Autodesk Fusion 360 part; units mm, degrees
(part 4 of 7)
sketch "Sketch83" plane through (0, 0, 14.6) normal (0, 0, -1) x (1, 0, 0)
  line L0 (95.9, -25.9) -> (101.9, -25.9)
  line L1 (95.9, -24.9) -> (95.9, -25.9)
  line L2 (126.4, -65.1) -> (125.4, -65.1)
  line L3 (106.4, -85.1) -> (106.4, -84.1)
  line L4 (106.4, -75.1) -> (106.4, -72.4023)
  line L5 (113.7023, -65.1) -> (116.4, -65.1)
  line L6 (116.4, -65.1) -> (113.7023, -65.1)
  line L7 (113.7023, -65.1) -> (114.7023, -65.1)
  line L8 (113.7023, -65.1) -> (114.7023, -65.1)
  line L9 (124.3722, -66.1) -> (115.1419, -66.1)
  line L10 (125.4, -65.1) -> (125.4, -59.1)
  line L11 (124.4, -65.1) -> (124.4, -60.1)
  line L12 (125.4, -59.1) -> (124.4, -59.1)
  arc A0 (106.4, -84.1) -> (125.4, -65.1) centre (106.4, -65.1) ccw
  arc A1 (106.4, -72.4023) -> (113.7023, -65.1) centre (106.4, -65.1) ccw
  arc A2 (109.2557, -72.8958) -> (114.1671, -68.0326) centre (106.4, -65.1) ccw
  line L13 (125.4, -65.1) -> (126.4, -65.1)
  line L14 (106.4, -73.4023) -> (106.4, -72.4023)
  line L15 (107.4, -74.049) -> (107.4, -83.0722)
  line L16 (106.4, -84.1) -> (100.4, -84.1)
  line L17 (100.4, -84.1) -> (100.4, -83.1)
  line L18 (101.4, -83.1) -> (106.4, -83.1)
  line L19 (106.4, -85.1) -> (106.4, -84.1)
  line L20 (100.4, -83.1) -> (106.4, -77.1)
  line L21 (101.4, -83.1) -> (108.8853, -83.1) construction
  line L22 (101.4, -83.1) -> (106.4, -78.1)
  line L23 (101.4, -83.1) -> (108.4711, -83.1) construction
  line L24 (106.4, -83.1) -> (106.4, -78.1)
  line L25 (106.4, -77.1) -> (106.4, -72.4023)
  line L26 (106.4, -83.1) -> (106.4, -78.1)
  line L27 (106.4, -77.1) -> (106.4, -75.1)
  line L28 (124.4, -59.1) -> (118.4, -65.1)
  line L29 (124.4, -59.1) -> (132.8853, -59.1) construction
  line L30 (119.4, -65.1) -> (124.4, -60.1)
  line L31 (119.4, -65.1) -> (126.4711, -65.1) construction
  line L32 (113.7023, -65.1) -> (118.4, -65.1)
  line L33 (119.4, -65.1) -> (124.4, -65.1)
  line L34 (124.4, -65.1) -> (119.4, -65.1)
  line L35 (118.4, -65.1) -> (114.7023, -65.1)
  line L36 (115.1419, -66.1) -> (125.3631, -66.1) construction
  line L37 (115.1419, -66.1) -> (122.396, -73.3541)
  line L38 (115.1419, -66.1) -> (125.8031, -66.1) construction
  line L39 (115.1106, -67.0687) -> (121.5189, -73.477)
  line L40 (121.5189, -73.477) -> (115.1106, -67.0687)
  arc A3 (122.396, -73.3541) -> (124.3722, -66.1) centre (106.4, -65.1) ccw
  line L41 (110.8485, -77.4975) -> (107.4, -74.049)
  line L42 (111.5557, -76.7904) -> (108.6326, -73.8674)
  line L43 (108.6326, -73.8674) -> (114.9008, -80.1355)
  line L44 (107.4, -74.049) -> (114.517, -81.166)
  arc A4 (107.4, -83.0722) -> (114.517, -81.166) centre (106.4, -65.1) ccw
  arc A5 (115.9173, -80.3781) -> (121.7571, -74.4894) centre (106.4, -65.1) ccw
  line L45 (115.7249, -77.2044) -> (115.9173, -80.3781)
  line L46 (114.7267, -77.2649) -> (114.9008, -80.1355)
  line L47 (117.5062, -74.2879) -> (121.7571, -74.4894)
  line L48 (117.5535, -73.2891) -> (121.5189, -73.477)
  line L49 (121.7571, -74.4894) -> (115.5425, -74.1949)
  line L50 (114.5378, -74.1472) -> (108.6326, -73.8674)
  line L51 (121.5189, -73.477) -> (115.4816, -73.1909)
  line L52 (114.4769, -73.1432) -> (109.2557, -72.8958)
  line L53 (115.9173, -80.3781) -> (115.5425, -74.1949)
  line L54 (115.4816, -73.1909) -> (115.1106, -67.0687)
  line L55 (114.9008, -80.1355) -> (114.5378, -74.1472)
  line L56 (114.4769, -73.1432) -> (114.1671, -68.0326)
  line L57 (27.2, 4.5) -> (66.7, 4.5)
  line L58 (46.95, 4.5) -> (46.95, -21.9501) construction
  line L59 (-13.5, -74.049) -> (-20.617, -81.166)
  line L60 (-14.7326, -73.8674) -> (-21.0008, -80.1355)
  circle A6 centre (-16.25, -62.1) radius 2.5
  line L61 (-12.5, -77.1) -> (-12.5, -75.1)
  arc A7 (-20.2671, -68.0326) -> (-15.3557, -72.8958) centre (-12.5, -65.1) ccw
  line L62 (-12.5, -73.4023) -> (-12.5, -72.4023)
  line L63 (-22.0173, -80.3781) -> (-21.6425, -74.1949)
  line L64 (-31.5, -59.1) -> (-30.5, -59.1)
  line L65 (-21.2419, -66.1) -> (-31.9031, -66.1) construction
  line L66 (-16.9485, -77.4975) -> (-13.5, -74.049)
  line L67 (-22.5, -65.1) -> (-19.8023, -65.1)
  line L68 (-20.5769, -73.1432) -> (-20.2671, -68.0326)
  arc A8 (-32.5, -65.1) -> (-12.5, -85.1) centre (-12.5, -65.1) ccw
  line L69 (-20.5769, -73.1432) -> (-15.3557, -72.8958)
  arc A9 (-19.8023, -65.1) -> (-12.5, -72.4023) centre (-12.5, -65.1) ccw
  arc A10 (-31.5, -65.1) -> (-12.5, -84.1) centre (-12.5, -65.1) ccw
  line L70 (-20.6378, -74.1472) -> (-14.7326, -73.8674)
  arc A11 (-20.617, -81.166) -> (-13.5, -83.0722) centre (-12.5, -65.1) ccw
  line L71 (-12.5, -85.1) -> (-12.5, -84.1)
  line L72 (-21.2106, -67.0687) -> (-27.6189, -73.477)
  line L73 (-25.5, -65.1) -> (-30.5, -65.1)
  line L74 (-19.8023, -65.1) -> (-24.5, -65.1)
  line L75 (-27.8571, -74.4894) -> (-21.6425, -74.1949)
  line L76 (-25.5, -65.1) -> (-30.5, -60.1)
  line L77 (-19.8023, -65.1) -> (-20.8023, -65.1)
  line L78 (-30.4722, -66.1) -> (-21.2419, -66.1)
  arc A12 (-27.8571, -74.4894) -> (-22.0173, -80.3781) centre (-12.5, -65.1) ccw
  arc A13 (-30.4722, -66.1) -> (-28.496, -73.3541) centre (-12.5, -65.1) ccw
  line L79 (-21.2419, -66.1) -> (-31.4631, -66.1) construction
  line L80 (-7.5, -83.1) -> (-14.5711, -83.1) construction
  line L81 (-13.5, -74.049) -> (-13.5, -83.0722)
  line L82 (-25.5, -65.1) -> (-32.5711, -65.1) construction
  line L83 (-30.5, -65.1) -> (-30.5, -60.1)
  line L84 (-6.5, -83.1) -> (-12.5, -77.1)
  line L85 (-21.0008, -80.1355) -> (-20.6378, -74.1472)
  line L86 (-12.5, -75.1) -> (-12.5, -72.4023)
  line L87 (-23.6062, -74.2879) -> (-27.8571, -74.4894)
  line L88 (-19.8023, -65.1) -> (-22.5, -65.1)
  line L89 (-31.5, -65.1) -> (-32.5, -65.1)
  line L90 (-12.5, -83.1) -> (-12.5, -78.1)
  line L91 (-17.6557, -76.7904) -> (-14.7326, -73.8674)
  line L92 (-7.5, -83.1) -> (-14.9853, -83.1) construction
  line L93 (-7.5, -83.1) -> (-12.5, -83.1)
  line L94 (-6.5, -84.1) -> (-6.5, -83.1)
  line L95 (-24.5, -65.1) -> (-20.8023, -65.1)
  line L96 (-12.5, -85.1) -> (-12.5, -84.1)
  line L97 (-21.8249, -77.2044) -> (-22.0173, -80.3781)
  line L98 (-12.5, -77.1) -> (-12.5, -72.4023)
  line L99 (-12.5, -84.1) -> (-6.5, -84.1)
  line L100 (-7.5, -83.1) -> (-12.5, -78.1)
  line L101 (-12.5, -83.1) -> (-12.5, -78.1)
  line L102 (-27.6189, -73.477) -> (-21.2106, -67.0687)
  line L103 (-20.8267, -77.2649) -> (-21.0008, -80.1355)
  line L104 (-30.5, -65.1) -> (-25.5, -65.1)
  line L105 (-30.5, -59.1) -> (-38.9853, -59.1) construction
  line L106 (-21.5816, -73.1909) -> (-21.2106, -67.0687)
  line L107 (-23.6535, -73.2891) -> (-27.6189, -73.477)
  line L108 (-32.5, -65.1) -> (-31.5, -65.1)
  line L109 (-27.6189, -73.477) -> (-21.5816, -73.1909)
  line L110 (-30.5, -59.1) -> (-24.5, -65.1)
  line L111 (-19.8023, -65.1) -> (-20.8023, -65.1)
  line L112 (-31.5, -65.1) -> (-31.5, -59.1)
  line L113 (-21.2419, -66.1) -> (-28.496, -73.3541)
  line L114 (101.9, -25.9) -> (101.9, -24.9)
  line L115 (101.9, -24.9) -> (95.9, -24.9)
  dimension "d560" = 1
  dimension "d561" = 1
  dimension "d562" = 1
  dimension "d563" = 1
  dimension "d566" = 6
  dimension "d567" = 6
  dimension "d569" = 6
  dimension "d570" = 1
  dimension "d571" = 45
  dimension "d572" = 1
  dimension "d573" = 45
  dimension "d574" = 135
  dimension "d575" = 1
  dimension "d576" = 45
  dimension "d580" = 45
  dimension "d583" = 1
  dimension "d585" = 1
  constraint parallel L4 L19
  constraint parallel L5 L7
  constraint concentric A1 A2
  constraint perpendicular L10 L32
  constraint coincident L14.start L19
  constraint coincident L4.end L19
  constraint collinear L13 L32
  constraint coincident L5.end L32
  constraint parallel L14 L19
  constraint perpendicular L3 L16
  constraint perpendicular L16 L17
  constraint collinear L19 L24
  constraint coincident L4.start L19
  constraint horizontal L21
  constraint coincident L20.end L26
  constraint horizontal L23
  constraint collinear L24 L25
  constraint collinear L26 L27
  constraint horizontal L29
  constraint horizontal L31
  constraint collinear L32 L33
  constraint collinear L34 L35
  constraint horizontal L36
  constraint horizontal L38
  constraint parallel L39 L40
  constraint concentric A3 A4
  constraint parallel L42 L43
  constraint parallel L41 L44
  constraint concentric A4 A5
  constraint parallel L46 L55
  constraint parallel L48 L51
  constraint collinear L49 L50
  constraint coincident L52.start L55
  constraint collinear L51 L52
  constraint coincident L51.end L53
  constraint collinear L53 L54
  constraint collinear L55 L56
  constraint midpoint L57 L58.start
  constraint perpendicular L57 L58
  constraint symmetric L3.start L58 A8.end
  constraint symmetric L2.start L58 A8.start
  constraint symmetric L2.end L58 A10.start
  constraint symmetric L3.end L58 A10.end
  constraint symmetric L18.end L58 L90.start
  constraint symmetric L4.start L58 L61.end
  constraint symmetric L5.end L58 L67.start
  constraint symmetric L5.start L58 L67.end
  constraint symmetric L7.end L58 L77.end
  constraint symmetric L11.start L58 L73.end
  constraint symmetric L10.end L58 L64.start
  constraint symmetric L12.end L58 L64.end
  constraint symmetric A0 L58 A10
  constraint symmetric L14.start L58 L62.start
  constraint symmetric L4.end L58 L62.end
  constraint symmetric A1 L58 A9
  constraint symmetric A2 L58 A7
  constraint symmetric L9.start L58 L78.start
  constraint symmetric L15.end L58 A11.end
  constraint symmetric L16.end L58 L94.start
  constraint symmetric L17.end L58 L84.start
  constraint symmetric L20.end L58 L61.start
  constraint symmetric L21.end L58 L92.end
  constraint symmetric L18.start L58 L80.start
  constraint symmetric L22.end L58 L90.end
  constraint symmetric L23.end L58 L80.end
  constraint symmetric L28.end L58 L74.end
  constraint symmetric L29.end L58 L105.end
  constraint symmetric L30.start L58 L73.start
  constraint symmetric L11.end L58 L76.end
  constraint symmetric L31.end L58 L82.end
  constraint symmetric L36.end L58 L79.end
  constraint symmetric L9.end L58 L65.start
  constraint symmetric L38.end L58 L65.end
  constraint symmetric L37.end L58 A13.end
  constraint symmetric A3 L58 A13
  constraint symmetric L42.start L58 L91.start
  constraint symmetric L41.start L58 L66.start
  constraint symmetric L44.end L58 L59.end
  constraint symmetric A4 L58 A11
  constraint symmetric A5 L58 A12
  constraint symmetric L15.start L58 L59.start
  constraint symmetric L46.start L58 L103.start
  constraint symmetric L45.start L58 L97.start
  constraint symmetric L47.start L58 L87.start
  constraint symmetric L48.start L58 L107.start
  constraint symmetric L43.end L58 L60.end
  constraint symmetric A5.start L58 L63.start
  constraint symmetric L49.end L58 L63.end
  constraint symmetric L52.start L58 L68.start
  constraint symmetric L50.start L58 L70.start
  constraint symmetric L51.end L58 L106.start
  constraint symmetric A2.end L58 A7.start
  constraint symmetric L39.start L58 L72.start
  constraint symmetric L42.end L58 L60.start
  constraint symmetric A2.start L58 A7.end
  constraint symmetric A5.end L58 L75.start
  constraint symmetric L39.end L58 L72.end
  measures "d560" distance of L2.start L2.end
  measures "d561" distance of L3.start L3.end
  measures "d562" distance of L3.end L18.end
  measures "d563" distance of L5.start L7.end
  measures "d566" distance of L2.end L10.end
  measures "d567" distance of L11.start L12.end
  measures "d569" distance of L3.end L16.end
  measures "d570" distance of L16.end L17.end
  measures "d571" angle of L20 L21
  measures "d572" distance of L17.end L18.start
  measures "d573" angle of L22 L23
  measures "d574" angle of L28 L29
  measures "d575" distance of L28.end L30.start
  measures "d576" angle of L30 L31
  measures "d580" angle of L37 L38
  measures "d583" distance of L42.start L41.start
  measures "d585" distance of L46.start L45.start
extrude "Extrude70" add sketch "Sketch83" along normal blind 1 contours L4 L5 L6 L7 L8 L10 L12 A0 A1 L14 L16 L17 L20 L25 L27 L28 L32 L35 | L61 L62 L64 L67 A9 A10 L74 L77 L84 L86 L88 L94 L95 L98 L99 L110 L111 L112 bodies 3 6
sketch "Sketch86" plane through (0, 0, 15.6) normal (0, 0, 1) x (-1, 0, 0)
  line L0 (29.1144, 32.8) -> (-123.0144, 32.8)
  arc A0 (-123.0144, 32.8) -> (-126.4, 25.3) centre (-116.4, 25.3) ccw
  line L1 (-126.4, 25.3) -> (-126.4, -65.1)
  arc A1 (-126.4, -65.1) -> (-106.4, -85.1) centre (-106.4, -65.1) ccw
  line L2 (-106.4, -85.1) -> (12.5, -85.1)
  arc A2 (12.5, -85.1) -> (32.5, -65.1) centre (12.5, -65.1) ccw
  line L3 (32.5, -65.1) -> (32.5, -25.2)
  line L4 (32.5, -25.2) -> (32.5, 25.3)
  arc A3 (32.5, 25.3) -> (29.1144, 32.8) centre (22.5, 25.3) ccw
  line L5 (13, -32.2) -> (19.5, -32.2)
  line L6 (19.5, -32.2) -> (19.5, -38.2)
  line L7 (19.5, -38.2) -> (25.5, -38.2)
  line L8 (25.5, -38.2) -> (25.5, -44.7)
  line L9 (25.5, -44.7) -> (19.5, -44.7)
  line L10 (19.5, -44.7) -> (19.5, -50.7)
  line L11 (19.5, -50.7) -> (13, -50.7)
  line L12 (13, -50.7) -> (13, -44.7)
  line L13 (13, -44.7) -> (7, -44.7)
  line L14 (7, -44.7) -> (7, -38.2)
  line L15 (7, -38.2) -> (13, -38.2)
  line L16 (13, -38.2) -> (13, -32.2)
  line L17 (-34.2, 32.4) -> (-34.2, 30.4)
  line L18 (-34.2, 30.4) -> (-27.2, 30.4)
  line L19 (-27.2, 30.4) -> (-27.2, 10)
  arc A4 (-29.2, 8) -> (-27.2, 10) centre (-29.2, 10) ccw
  line L20 (-29.2, 8) -> (-64.7, 8)
  arc A5 (-66.7, 10) -> (-64.7, 8) centre (-64.7, 10) ccw
  line L21 (-66.7, 10) -> (-66.7, 30.4)
  line L22 (-66.7, 30.4) -> (-59.7, 30.4)
  line L23 (-59.7, 30.4) -> (-59.7, 32.4)
  line L24 (-59.7, 32.4) -> (-34.2, 32.4)
  arc A6 (5, 10.7) -> (5.0004, 12.7) centre (5, 11.7) ccw
  line L25 (5, 10.7) -> (-5, 10.7)
  arc A7 (-5.0004, 12.7) -> (-5, 10.7) centre (-5, 11.7) ccw
  line L26 (-5.0004, 12.7) -> (5.0004, 12.7)
  arc A8 (5.0004, 26.7) -> (5, 28.7) centre (5, 27.7) ccw
  line L27 (5.0004, 26.7) -> (-4.9996, 26.7)
  arc A9 (-5, 28.7) -> (-4.9996, 26.7) centre (-5, 27.7) ccw
  line L28 (-5, 28.7) -> (5, 28.7)
  line L29 (-8.1652, 24.7) -> (8.1652, 24.7)
  arc A10 (8.1652, 22.7) -> (8.1652, 24.7) centre (8.1652, 23.7) ccw
  line L30 (8.1652, 22.7) -> (-8.1652, 22.7)
  arc A11 (-8.1652, 24.7) -> (-8.1652, 22.7) centre (-8.1652, 23.7) ccw
  arc A12 (9, 18.7) -> (9, 20.7) centre (9, 19.7) ccw
  line L31 (9, 18.7) -> (-9, 18.7)
  arc A13 (-9, 20.7) -> (-9, 18.7) centre (-9, 19.7) ccw
  line L32 (-9, 20.7) -> (9, 20.7)
  line L33 (8.1652, 14.7) -> (-8.1652, 14.7)
  arc A14 (-8.1652, 16.7) -> (-8.1652, 14.7) centre (-8.1652, 15.7) ccw
  line L34 (-8.1652, 16.7) -> (8.1652, 16.7)
  arc A15 (8.1652, 14.7) -> (8.1652, 16.7) centre (8.1652, 15.7) ccw
  arc A16 (-102.9, 20.7) -> (-102.9, 18.7) centre (-102.9, 19.7) ccw
  line L35 (-102.9, 20.7) -> (-84.9, 20.7)
  arc A17 (-84.9, 18.7) -> (-84.9, 20.7) centre (-84.9, 19.7) ccw
  line L36 (-84.9, 18.7) -> (-102.9, 18.7)
  arc A18 (-98.9, 28.7) -> (-98.9004, 26.7) centre (-98.9, 27.7) ccw
  line L37 (-98.9, 28.7) -> (-88.9, 28.7)
  arc A19 (-88.8996, 26.7) -> (-88.9, 28.7) centre (-88.9, 27.7) ccw
  line L38 (-88.8996, 26.7) -> (-98.9004, 26.7)
  arc A20 (-102.0652, 24.7) -> (-102.0652, 22.7) centre (-102.0652, 23.7) ccw
  line L39 (-102.0652, 24.7) -> (-85.7348, 24.7)
  arc A21 (-85.7348, 22.7) -> (-85.7348, 24.7) centre (-85.7348, 23.7) ccw
  line L40 (-85.7348, 22.7) -> (-102.0652, 22.7)
  line L41 (-85.7348, 14.7) -> (-102.0652, 14.7)
  arc A22 (-102.0652, 16.7) -> (-102.0652, 14.7) centre (-102.0652, 15.7) ccw
  line L42 (-102.0652, 16.7) -> (-85.7348, 16.7)
  arc A23 (-85.7348, 14.7) -> (-85.7348, 16.7) centre (-85.7348, 15.7) ccw
  line L43 (-98.8996, 12.7) -> (-88.8996, 12.7)
  arc A24 (-88.9, 10.7) -> (-88.8996, 12.7) centre (-88.9, 11.7) ccw
  line L44 (-88.9, 10.7) -> (-98.9, 10.7)
  arc A25 (-98.8996, 12.7) -> (-98.9, 10.7) centre (-98.9, 11.7) ccw
  arc A26 (-46.45, -79.6) -> (-47.45, -79.6) centre (-46.95, -79.6) ccw
  line L45 (-46.45, -79.6) -> (-45.65, -79.6)
  arc A27 (-45.65, -80.6) -> (-45.65, -79.6) centre (-45.65, -80.1) ccw
  line L46 (-45.65, -80.6) -> (-46.45, -80.6)
  arc A28 (-47.45, -80.6) -> (-46.45, -80.6) centre (-46.95, -80.6) ccw
  line L47 (-47.45, -80.6) -> (-48.25, -80.6)
  arc A29 (-48.25, -79.6) -> (-48.25, -80.6) centre (-48.25, -80.1) ccw
  line L48 (-48.25, -79.6) -> (-47.45, -79.6)
  circle A30 centre (-110.15, -48.95) radius 3.85
  circle A31 centre (-117.65, -41.45) radius 3.85
  circle A32 centre (-102.65, -41.45) radius 3.85
  circle A33 centre (-110.15, -33.95) radius 3.85
  circle A34 centre (-117.6453, -56.4453) radius 2.35
  circle A35 centre (-102.6547, -56.4453) radius 2.35
  line L49 (0, 4.1) -> (0, -75.1)
  line L50 (0, -75.1) -> (-93.9, -75.1)
  line L51 (-93.9, -75.1) -> (-93.9, 4.1)
  line L52 (-93.9, 4.1) -> (0, 4.1)
  circle A36 centre (10.8119, -62.3239) radius 1.5
  dimension "d597" = 3
  measures "d597" diameter of A36
sketch "Sketch87" plane through (0, 0, 14.6) normal (0, 0, -1) x (1, 0, 0)
  arc A0 (-31.5, -65.1) -> (-12.5, -84.1) centre (-12.5, -65.1) ccw
  line L0 (-31.5, -65.1) -> (-31.5, -59.1)
  line L1 (-31.5, -59.1) -> (-30.5, -59.1)
  line L2 (-30.5, -59.1) -> (-24.5, -65.1)
  line L3 (-24.5, -65.1) -> (-19.8023, -65.1)
  arc A1 (-19.8023, -65.1) -> (-12.5, -72.4023) centre (-12.5, -65.1) ccw
  line L4 (-12.5, -72.4023) -> (-12.5, -77.1)
  line L5 (-12.5, -77.1) -> (-6.5, -83.1)
  line L6 (-6.5, -83.1) -> (-6.5, -84.1)
  line L7 (-6.5, -84.1) -> (-12.5, -84.1)
  line L8 (-14, -21.7213) -> (-14, -21.5571)
  arc A2 (-18.6299, -19.9) -> (-14, -21.5571) centre (-16.1626, -20.3028) ccw
  line L9 (-18.6299, -19.9) -> (-18.6563, -19.9)
  arc A3 (-18.6098, -19.7916) -> (-18.6563, -19.9) centre (-16.3363, -20.8316) ccw
  arc A4 (-13.8891, -21.3427) -> (-18.6098, -19.7916) centre (-16.1626, -20.3028) ccw
  arc A5 (-14, -21.7213) -> (-13.8891, -21.3427) centre (-16.3363, -20.8316) ccw
  circle A6 centre (-16.25, -62.1) radius 2.5
  arc A7 (-9.5307, -48.3426) -> (-9.5307, -34.5574) centre (-10.1676, -41.45) ccw
  arc A8 (-22.9827, -48.1827) -> (-9.5307, -48.3426) centre (-16.25, -47.7) ccw
  arc A9 (-22.9827, -34.7173) -> (-22.9827, -48.1827) centre (-22.5, -41.45) ccw
  arc A10 (-9.5307, -34.5574) -> (-22.9827, -34.7173) centre (-16.25, -35.2) ccw
  line L10 (-2, -24.9) -> (-8, -24.9)
  line L11 (-8, -24.9) -> (-8, -7.9)
  line L12 (-8, -7.9) -> (-13, -7.9)
  line L13 (-13, -7.9) -> (-13, -13.9)
  line L14 (-13, -13.9) -> (-25, -13.9)
  line L15 (-25, -13.9) -> (-25, -24.9)
  line L16 (-25, -24.9) -> (-30.5, -24.9)
  line L17 (-30.5, -24.9) -> (-30.5, -25.9)
  line L18 (-30.5, -25.9) -> (-31.5, -25.9)
  line L19 (-31.5, -25.9) -> (-31.5, 4.1)
  line L20 (-31.5, 4.1) -> (-32.5, 4.1)
  line L21 (-32.5, 4.1) -> (-32.5, -25.2)
  line L22 (-32.5, -25.2) -> (-32.5, -65.1)
  arc A11 (-32.5, -65.1) -> (-12.5, -85.1) centre (-12.5, -65.1) ccw
  line L23 (-12.5, -85.1) -> (-2, -85.1)
  line L24 (-2, -85.1) -> (-2, -24.9)
  line L25 (-5, -75) -> (-6, -75)
  line L26 (-6, -75) -> (-6, -57)
  line L27 (-6, -57) -> (-5, -57)
  line L28 (-5, -57) -> (-5, -75)
  line L29 (-27.5, -62.1) -> (-28.5, -62.1)
  line L30 (-28.5, -62.1) -> (-28.5, -52.1)
  line L31 (-28.5, -52.1) -> (-27.5, -52.1)
  line L32 (-27.5, -52.1) -> (-27.5, -62.1)
  dimension "d602" = 1
  dimension "d603" = 10
  constraint horizontal L25
  constraint vertical L26
  constraint horizontal L27
  constraint vertical L28
  constraint horizontal L29
  constraint vertical L30
  constraint horizontal L31
  constraint vertical L32
  constraint midpoint L2 L29.start
  measures "d602" distance of L29.start L29.end
  measures "d603" distance of L29.start L31.end
extrude "Extrude72" add sketch "Sketch87" along normal blind 1 contours L2 L30 L31 L32 | L25 L26 L27 L28 bodies 3 6 8
extrude "Extrude73" cut sketch "Sketch86" against normal blind 1 contours A36 bodies 3
sketch "Sketch88" plane through (0, 0, 15.6) normal (0, 0, 1) x (-1, 0, 0)
  circle A0 centre (10.8119, -62.3239) radius 1.5
  line L0 (29.1144, 32.8) -> (-123.0144, 32.8)
  arc A1 (-123.0144, 32.8) -> (-126.4, 25.3) centre (-116.4, 25.3) ccw
  line L1 (-126.4, 25.3) -> (-126.4, -65.1)
  arc A2 (-126.4, -65.1) -> (-106.4, -85.1) centre (-106.4, -65.1) ccw
  line L2 (-106.4, -85.1) -> (12.5, -85.1)
  arc A3 (12.5, -85.1) -> (32.5, -65.1) centre (12.5, -65.1) ccw
  line L3 (32.5, -65.1) -> (32.5, -25.2)
  line L4 (32.5, -25.2) -> (32.5, 25.3)
  arc A4 (32.5, 25.3) -> (29.1144, 32.8) centre (22.5, 25.3) ccw
  line L5 (13, -32.2) -> (19.5, -32.2)
  line L6 (19.5, -32.2) -> (19.5, -38.2)
  line L7 (19.5, -38.2) -> (25.5, -38.2)
  line L8 (25.5, -38.2) -> (25.5, -44.7)
  line L9 (25.5, -44.7) -> (19.5, -44.7)
  line L10 (19.5, -44.7) -> (19.5, -50.7)
  line L11 (19.5, -50.7) -> (13, -50.7)
  line L12 (13, -50.7) -> (13, -44.7)
  line L13 (13, -44.7) -> (7, -44.7)
  line L14 (7, -44.7) -> (7, -38.2)
  line L15 (7, -38.2) -> (13, -38.2)
  line L16 (13, -38.2) -> (13, -32.2)
  line L17 (-34.2, 32.4) -> (-34.2, 30.4)
  line L18 (-34.2, 30.4) -> (-27.2, 30.4)
  line L19 (-27.2, 30.4) -> (-27.2, 10)
  arc A5 (-29.2, 8) -> (-27.2, 10) centre (-29.2, 10) ccw
  line L20 (-29.2, 8) -> (-64.7, 8)
  arc A6 (-66.7, 10) -> (-64.7, 8) centre (-64.7, 10) ccw
  line L21 (-66.7, 10) -> (-66.7, 30.4)
  line L22 (-66.7, 30.4) -> (-59.7, 30.4)
  line L23 (-59.7, 30.4) -> (-59.7, 32.4)
  line L24 (-59.7, 32.4) -> (-34.2, 32.4)
  arc A7 (5, 10.7) -> (5.0004, 12.7) centre (5, 11.7) ccw
  line L25 (5, 10.7) -> (-5, 10.7)
  arc A8 (-5.0004, 12.7) -> (-5, 10.7) centre (-5, 11.7) ccw
  line L26 (-5.0004, 12.7) -> (5.0004, 12.7)
  arc A9 (5.0004, 26.7) -> (5, 28.7) centre (5, 27.7) ccw
  line L27 (5.0004, 26.7) -> (-4.9996, 26.7)
  arc A10 (-5, 28.7) -> (-4.9996, 26.7) centre (-5, 27.7) ccw
  line L28 (-5, 28.7) -> (5, 28.7)
  line L29 (-8.1652, 24.7) -> (8.1652, 24.7)
  arc A11 (8.1652, 22.7) -> (8.1652, 24.7) centre (8.1652, 23.7) ccw
  line L30 (8.1652, 22.7) -> (-8.1652, 22.7)
  arc A12 (-8.1652, 24.7) -> (-8.1652, 22.7) centre (-8.1652, 23.7) ccw
  arc A13 (9, 18.7) -> (9, 20.7) centre (9, 19.7) ccw
  line L31 (9, 18.7) -> (-9, 18.7)
  arc A14 (-9, 20.7) -> (-9, 18.7) centre (-9, 19.7) ccw
  line L32 (-9, 20.7) -> (9, 20.7)
  line L33 (8.1652, 14.7) -> (-8.1652, 14.7)
  arc A15 (-8.1652, 16.7) -> (-8.1652, 14.7) centre (-8.1652, 15.7) ccw
  line L34 (-8.1652, 16.7) -> (8.1652, 16.7)
  arc A16 (8.1652, 14.7) -> (8.1652, 16.7) centre (8.1652, 15.7) ccw
  arc A17 (-102.9, 20.7) -> (-102.9, 18.7) centre (-102.9, 19.7) ccw
  line L35 (-102.9, 20.7) -> (-84.9, 20.7)
  arc A18 (-84.9, 18.7) -> (-84.9, 20.7) centre (-84.9, 19.7) ccw
  line L36 (-84.9, 18.7) -> (-102.9, 18.7)
  arc A19 (-98.9, 28.7) -> (-98.9004, 26.7) centre (-98.9, 27.7) ccw
  line L37 (-98.9, 28.7) -> (-88.9, 28.7)
  arc A20 (-88.8996, 26.7) -> (-88.9, 28.7) centre (-88.9, 27.7) ccw
  line L38 (-88.8996, 26.7) -> (-98.9004, 26.7)
  arc A21 (-102.0652, 24.7) -> (-102.0652, 22.7) centre (-102.0652, 23.7) ccw
  line L39 (-102.0652, 24.7) -> (-85.7348, 24.7)
  arc A22 (-85.7348, 22.7) -> (-85.7348, 24.7) centre (-85.7348, 23.7) ccw
  line L40 (-85.7348, 22.7) -> (-102.0652, 22.7)
  line L41 (-85.7348, 14.7) -> (-102.0652, 14.7)
  arc A23 (-102.0652, 16.7) -> (-102.0652, 14.7) centre (-102.0652, 15.7) ccw
  line L42 (-102.0652, 16.7) -> (-85.7348, 16.7)
  arc A24 (-85.7348, 14.7) -> (-85.7348, 16.7) centre (-85.7348, 15.7) ccw
  line L43 (-98.8996, 12.7) -> (-88.8996, 12.7)
  arc A25 (-88.9, 10.7) -> (-88.8996, 12.7) centre (-88.9, 11.7) ccw
  line L44 (-88.9, 10.7) -> (-98.9, 10.7)
  arc A26 (-98.8996, 12.7) -> (-98.9, 10.7) centre (-98.9, 11.7) ccw
  arc A27 (-46.45, -79.6) -> (-47.45, -79.6) centre (-46.95, -79.6) ccw
  line L45 (-46.45, -79.6) -> (-45.65, -79.6)
  arc A28 (-45.65, -80.6) -> (-45.65, -79.6) centre (-45.65, -80.1) ccw
  line L46 (-45.65, -80.6) -> (-46.45, -80.6)
  arc A29 (-47.45, -80.6) -> (-46.45, -80.6) centre (-46.95, -80.6) ccw
  line L47 (-47.45, -80.6) -> (-48.25, -80.6)
  arc A30 (-48.25, -79.6) -> (-48.25, -80.6) centre (-48.25, -80.1) ccw
  line L48 (-48.25, -79.6) -> (-47.45, -79.6)
  circle A31 centre (-110.15, -48.95) radius 3.85
  circle A32 centre (-117.65, -41.45) radius 3.85
  circle A33 centre (-102.65, -41.45) radius 3.85
  circle A34 centre (-110.15, -33.95) radius 3.85
  circle A35 centre (-117.6453, -56.4453) radius 2.35
  circle A36 centre (-102.6547, -56.4453) radius 2.35
  line L49 (0, 4.1) -> (0, -75.1)
  line L50 (0, -75.1) -> (-93.9, -75.1)
  line L51 (-93.9, -75.1) -> (-93.9, 4.1)
  line L52 (-93.9, 4.1) -> (0, 4.1)
  arc A37 (-47.4908, -77.2) -> (-46.4092, -77.2) centre (-46.95, -80.1) ccw
  line L53 (-46.95, -80.1) -> (-34.95, -80.1) construction
  line L54 (-34.95, -80.1) -> (-34.95, -78.1) construction
  line L55 (-34.95, -80.1) -> (-34.95, -82.1) construction
  line L56 (-34.95, -79.1) -> (-34.95, -81.1)
  line L57 (-34.95, -81.1) -> (-35.95, -81.1)
  line L58 (-35.95, -81.1) -> (-36.95, -80.1)
  line L59 (-35.95, -81.1) -> (-34.5358, -81.1) construction
  line L60 (-36.95, -80.1) -> (-37.95, -81.1)
  line L61 (-37.95, -81.1) -> (-38.95, -81.1)
  line L62 (-38.95, -81.1) -> (-38.95, -79.1)
  line L63 (-34.95, -79.1) -> (-35.95, -79.1)
  line L64 (-35.95, -79.1) -> (-35.95, -80.1)
  line L65 (-35.95, -80.1) -> (-36.95, -79.1)
  line L66 (-36.95, -79.1) -> (-37.95, -80.1)
  line L67 (-37.95, -80.1) -> (-37.95, -79.1)
  line L68 (-37.95, -79.1) -> (-38.95, -79.1)
  line L69 (-38.95, -81.1) -> (-39.55, -81.1) construction
  line L70 (-39.55, -81.1) -> (-39.55, -79.1)
  line L71 (-39.55, -79.1) -> (-40.55, -79.1)
  line L72 (-39.55, -81.1) -> (-40.55, -81.1)
  line L73 (-40.55, -81.1) -> (-40.55, -79.1)
  line L74 (-40.95, -80.1) -> (-41.05, -80.1) construction
  line L75 (-41.05, -80.1) -> (-42.05, -80.1)
  line L76 (-42.05, -80.1) -> (-42.05, -81.1) construction
  line L77 (-42.05, -81.1) -> (-42.05, -79.1) construction
  arc A38 (-42.05, -81.1) -> (-42.05, -79.1) centre (-42.05, -80.1) ccw
  line L78 (-42.05, -81.1) -> (-42.55, -81.1)
  line L79 (-42.05, -79.1) -> (-42.55, -79.1)
  line L80 (-42.55, -79.1) -> (-42.55, -79.6)
  line L81 (-42.55, -81.1) -> (-42.55, -80.6)
  line L82 (-42.05, -80.1) -> (-42.55, -80.1)
  arc A39 (-42.55, -80.6) -> (-42.55, -79.6) centre (-42.55, -80.1) ccw
  dimension "d604" = 12
  dimension "d605" = 2
  dimension "d606" = 2
  dimension "d607" = 1
  dimension "d608" = 135
  dimension "d609" = 1
  dimension "d610" = 1
  dimension "d611" = 0.6
  dimension "d612" = 1
  dimension "d613" = 0.1
  dimension "d614" = 1
  dimension "d615" = 0.5
  dimension "d616" = 0.5
  dimension "d617" = 0.5
  dimension "d618" = 0.5
  dimension "d619" = 0.5
  constraint coincident A37.centre L53.start
  constraint parallel L45 L53
  constraint perpendicular L53 L54
  constraint perpendicular L53 L55
  constraint midpoint L54 L56.start
  constraint midpoint L55 L56.end
  constraint perpendicular L55 L57
  constraint horizontal L59
  constraint coincident L53 L58.end
  constraint perpendicular L58 L60
  constraint parallel L53 L61
  constraint perpendicular L53 L62
  constraint perpendicular L54 L63
  constraint coincident L53 L64.end
  constraint perpendicular L53 L64
  constraint parallel L58 L65
  constraint coincident L53 L66.end
  constraint perpendicular L65 L66
  constraint perpendicular L53 L67
  constraint perpendicular L62 L68
  constraint perpendicular L62 L69
  constraint perpendicular L68 L70
  constraint perpendicular L70 L71
  constraint perpendicular L70 L72
  constraint perpendicular L71 L73
  constraint midpoint L53 L74.start
  constraint perpendicular L73 L74
  constraint parallel L53 L75
  constraint coincident L75.end L76.start
  constraint coincident L74.end A38
  constraint perpendicular L53 L76
  constraint perpendicular L53 L77
  constraint perpendicular L76 L78
  constraint perpendicular L77 L79
  constraint perpendicular L79 L80
  constraint perpendicular L78 L81
  constraint perpendicular L81 L82
  constraint coincident L82.end A39.centre
  constraint coincident L75.end A39
  measures "d604" distance of A37.centre L53.end
  measures "d605" distance of L53.end L54.end
  measures "d606" distance of L53.end L55.end
  measures "d607" distance of L56.end L57.end
  measures "d608" angle of L58 L59
  measures "d609" distance of L60.end L61.end
  measures "d610" distance of L56.start L63.end
  measures "d611" distance of L61.end L69.end
  measures "d612" distance of L70.end L71.end
  measures "d613" distance of L74.start L74.end
  measures "d614" distance of L74.end L75.end
  measures "d615" distance of L76.end L78.end
  measures "d616" distance of L77.end L79.end
  measures "d617" distance of L79.end L80.end
  measures "d618" distance of L78.end L81.end
  measures "d619" distance of L75.end L82.end
sketch "icon1" plane through (0, 0, 15.6) normal (0, 0, 1) x (-1, 0, 0)
  circle A0 centre (10.8119, -62.3239) radius 1.5
  line L0 (29.1144, 32.8) -> (-123.0144, 32.8)
  arc A1 (-123.0144, 32.8) -> (-126.4, 25.3) centre (-116.4, 25.3) ccw
  line L1 (-126.4, 25.3) -> (-126.4, -65.1)
  arc A2 (-126.4, -65.1) -> (-106.4, -85.1) centre (-106.4, -65.1) ccw
  line L2 (-106.4, -85.1) -> (12.5, -85.1)
  arc A3 (12.5, -85.1) -> (32.5, -65.1) centre (12.5, -65.1) ccw
  line L3 (32.5, -65.1) -> (32.5, -25.2)
  line L4 (32.5, -25.2) -> (32.5, 25.3)
  arc A4 (32.5, 25.3) -> (29.1144, 32.8) centre (22.5, 25.3) ccw
  line L5 (13, -32.2) -> (19.5, -32.2)
  line L6 (19.5, -32.2) -> (19.5, -38.2)
  line L7 (19.5, -38.2) -> (25.5, -38.2)
  line L8 (25.5, -38.2) -> (25.5, -44.7)
  line L9 (25.5, -44.7) -> (19.5, -44.7)
  line L10 (19.5, -44.7) -> (19.5, -50.7)
  line L11 (19.5, -50.7) -> (13, -50.7)
  line L12 (13, -50.7) -> (13, -44.7)
  line L13 (13, -44.7) -> (7, -44.7)
  line L14 (7, -44.7) -> (7, -38.2)
  line L15 (7, -38.2) -> (13, -38.2)
  line L16 (13, -38.2) -> (13, -32.2)
  line L17 (-34.2, 32.4) -> (-34.2, 30.4)
  line L18 (-34.2, 30.4) -> (-27.2, 30.4)
  line L19 (-27.2, 30.4) -> (-27.2, 10)
  arc A5 (-29.2, 8) -> (-27.2, 10) centre (-29.2, 10) ccw
  line L20 (-29.2, 8) -> (-64.7, 8)
  arc A6 (-66.7, 10) -> (-64.7, 8) centre (-64.7, 10) ccw
  line L21 (-66.7, 10) -> (-66.7, 30.4)
  line L22 (-66.7, 30.4) -> (-59.7, 30.4)
  line L23 (-59.7, 30.4) -> (-59.7, 32.4)
  line L24 (-59.7, 32.4) -> (-34.2, 32.4)
  arc A7 (5, 10.7) -> (5.0004, 12.7) centre (5, 11.7) ccw
  line L25 (5, 10.7) -> (-5, 10.7)
  arc A8 (-5.0004, 12.7) -> (-5, 10.7) centre (-5, 11.7) ccw
  line L26 (-5.0004, 12.7) -> (5.0004, 12.7)
  arc A9 (5.0004, 26.7) -> (5, 28.7) centre (5, 27.7) ccw
  line L27 (5.0004, 26.7) -> (-4.9996, 26.7)
  arc A10 (-5, 28.7) -> (-4.9996, 26.7) centre (-5, 27.7) ccw
  line L28 (-5, 28.7) -> (5, 28.7)
  line L29 (-8.1652, 24.7) -> (8.1652, 24.7)
  arc A11 (8.1652, 22.7) -> (8.1652, 24.7) centre (8.1652, 23.7) ccw
  line L30 (8.1652, 22.7) -> (-8.1652, 22.7)
  arc A12 (-8.1652, 24.7) -> (-8.1652, 22.7) centre (-8.1652, 23.7) ccw
  arc A13 (9, 18.7) -> (9, 20.7) centre (9, 19.7) ccw
  line L31 (9, 18.7) -> (-9, 18.7)
  arc A14 (-9, 20.7) -> (-9, 18.7) centre (-9, 19.7) ccw
  line L32 (-9, 20.7) -> (9, 20.7)
  line L33 (8.1652, 14.7) -> (-8.1652, 14.7)
  arc A15 (-8.1652, 16.7) -> (-8.1652, 14.7) centre (-8.1652, 15.7) ccw
  line L34 (-8.1652, 16.7) -> (8.1652, 16.7)
  arc A16 (8.1652, 14.7) -> (8.1652, 16.7) centre (8.1652, 15.7) ccw
  arc A17 (-102.9, 20.7) -> (-102.9, 18.7) centre (-102.9, 19.7) ccw
  line L35 (-102.9, 20.7) -> (-84.9, 20.7)
  arc A18 (-84.9, 18.7) -> (-84.9, 20.7) centre (-84.9, 19.7) ccw
  line L36 (-84.9, 18.7) -> (-102.9, 18.7)
  arc A19 (-98.9, 28.7) -> (-98.9004, 26.7) centre (-98.9, 27.7) ccw
  line L37 (-98.9, 28.7) -> (-88.9, 28.7)
  arc A20 (-88.8996, 26.7) -> (-88.9, 28.7) centre (-88.9, 27.7) ccw
  line L38 (-88.8996, 26.7) -> (-98.9004, 26.7)
  arc A21 (-102.0652, 24.7) -> (-102.0652, 22.7) centre (-102.0652, 23.7) ccw
  line L39 (-102.0652, 24.7) -> (-85.7348, 24.7)
  arc A22 (-85.7348, 22.7) -> (-85.7348, 24.7) centre (-85.7348, 23.7) ccw
  line L40 (-85.7348, 22.7) -> (-102.0652, 22.7)
  line L41 (-85.7348, 14.7) -> (-102.0652, 14.7)
  arc A23 (-102.0652, 16.7) -> (-102.0652, 14.7) centre (-102.0652, 15.7) ccw
  line L42 (-102.0652, 16.7) -> (-85.7348, 16.7)
  arc A24 (-85.7348, 14.7) -> (-85.7348, 16.7) centre (-85.7348, 15.7) ccw
  line L43 (-98.8996, 12.7) -> (-88.8996, 12.7)
  arc A25 (-88.9, 10.7) -> (-88.8996, 12.7) centre (-88.9, 11.7) ccw
  line L44 (-88.9, 10.7) -> (-98.9, 10.7)
  arc A26 (-98.8996, 12.7) -> (-98.9, 10.7) centre (-98.9, 11.7) ccw
  arc A27 (-46.45, -79.6) -> (-47.45, -79.6) centre (-46.95, -79.6) ccw
  line L45 (-46.45, -79.6) -> (-45.65, -79.6)
  arc A28 (-45.65, -80.6) -> (-45.65, -79.6) centre (-45.65, -80.1) ccw
  line L46 (-45.65, -80.6) -> (-46.45, -80.6)
  arc A29 (-47.45, -80.6) -> (-46.45, -80.6) centre (-46.95, -80.6) ccw
  line L47 (-47.45, -80.6) -> (-48.25, -80.6)
  arc A30 (-48.25, -79.6) -> (-48.25, -80.6) centre (-48.25, -80.1) ccw
  line L48 (-48.25, -79.6) -> (-47.45, -79.6)
  circle A31 centre (-110.15, -48.95) radius 3.85
  circle A32 centre (-117.65, -41.45) radius 3.85
  circle A33 centre (-102.65, -41.45) radius 3.85
  circle A34 centre (-110.15, -33.95) radius 3.85
  circle A35 centre (-117.6453, -56.4453) radius 2.35
  circle A36 centre (-102.6547, -56.4453) radius 2.35
  line L49 (0, 4.1) -> (0, -75.1)
  line L50 (0, -75.1) -> (-93.9, -75.1)
  line L51 (-93.9, -75.1) -> (-93.9, 4.1)
  line L52 (-93.9, 4.1) -> (0, 4.1)
  circle A37 centre (16, 30.9) radius 0.4
  line L53 (15.744, 30.5926) -> (16.4, 29.8)
  line L54 (16.4, 29.8) -> (16.5662, 29.9375)
  line L55 (16.5662, 29.9375) -> (16, 30.6217)
  line L56 (16.5662, 29.9375) -> (16.8018, 29.6528)
  line L57 (16.8018, 29.6528) -> (16.0141, 29.4807)
  line L58 (16.0141, 29.4807) -> (16.4, 29.8)
  line L59 (16.0919, 31.9806) -> (16.0919, 32.8)
  line L60 (16.0919, 32.8) -> (16.0919, 31.8676)
  line L61 (16.0919, 32.8) -> (17.2457, 31.2867)
  arc A38 (16.0919, 31.8676) -> (17.2457, 31.2867) centre (16.072, 30.3917) ccw
  constraint coincident A37 L53.start
  constraint perpendicular L53 L54
  constraint perpendicular L54 L55
  constraint perpendicular L54 L56
  constraint perpendicular L56 L58
  constraint coincident L0 L59.end
  constraint perpendicular L0 L59
  constraint perpendicular L0 L60
  constraint tangent L61 A38
sketch "icon2" plane through (0, 0, 15.6) normal (0, 0, 1) x (-1, 0, 0)
  circle A0 centre (10.8119, -62.3239) radius 1.5
  line L0 (29.1144, 32.8) -> (-123.0144, 32.8)
  arc A1 (-123.0144, 32.8) -> (-126.4, 25.3) centre (-116.4, 25.3) ccw
  line L1 (-126.4, 25.3) -> (-126.4, -65.1)
  arc A2 (-126.4, -65.1) -> (-106.4, -85.1) centre (-106.4, -65.1) ccw
  line L2 (-106.4, -85.1) -> (12.5, -85.1)
  arc A3 (12.5, -85.1) -> (32.5, -65.1) centre (12.5, -65.1) ccw
  line L3 (32.5, -65.1) -> (32.5, -25.2)
  line L4 (32.5, -25.2) -> (32.5, 25.3)
  arc A4 (32.5, 25.3) -> (29.1144, 32.8) centre (22.5, 25.3) ccw
  line L5 (13, -32.2) -> (19.5, -32.2)
  line L6 (19.5, -32.2) -> (19.5, -38.2)
  line L7 (19.5, -38.2) -> (25.5, -38.2)
  line L8 (25.5, -38.2) -> (25.5, -44.7)
  line L9 (25.5, -44.7) -> (19.5, -44.7)
  line L10 (19.5, -44.7) -> (19.5, -50.7)
  line L11 (19.5, -50.7) -> (13, -50.7)
  line L12 (13, -50.7) -> (13, -44.7)
  line L13 (13, -44.7) -> (7, -44.7)
  line L14 (7, -44.7) -> (7, -38.2)
  line L15 (7, -38.2) -> (13, -38.2)
  line L16 (13, -38.2) -> (13, -32.2)
  line L17 (-34.2, 32.4) -> (-34.2, 30.4)
  line L18 (-34.2, 30.4) -> (-27.2, 30.4)
  line L19 (-27.2, 30.4) -> (-27.2, 10)
  arc A5 (-29.2, 8) -> (-27.2, 10) centre (-29.2, 10) ccw
  line L20 (-29.2, 8) -> (-64.7, 8)
  arc A6 (-66.7, 10) -> (-64.7, 8) centre (-64.7, 10) ccw
  line L21 (-66.7, 10) -> (-66.7, 30.4)
  line L22 (-66.7, 30.4) -> (-59.7, 30.4)
  line L23 (-59.7, 30.4) -> (-59.7, 32.4)
  line L24 (-59.7, 32.4) -> (-34.2, 32.4)
  arc A7 (5, 10.7) -> (5.0004, 12.7) centre (5, 11.7) ccw
  line L25 (5, 10.7) -> (-5, 10.7)
  arc A8 (-5.0004, 12.7) -> (-5, 10.7) centre (-5, 11.7) ccw
  line L26 (-5.0004, 12.7) -> (5.0004, 12.7)
  arc A9 (5.0004, 26.7) -> (5, 28.7) centre (5, 27.7) ccw
  line L27 (5.0004, 26.7) -> (-4.9996, 26.7)
  arc A10 (-5, 28.7) -> (-4.9996, 26.7) centre (-5, 27.7) ccw
  line L28 (-5, 28.7) -> (5, 28.7)
  line L29 (-8.1652, 24.7) -> (8.1652, 24.7)
  arc A11 (8.1652, 22.7) -> (8.1652, 24.7) centre (8.1652, 23.7) ccw
  line L30 (8.1652, 22.7) -> (-8.1652, 22.7)
  arc A12 (-8.1652, 24.7) -> (-8.1652, 22.7) centre (-8.1652, 23.7) ccw
  arc A13 (9, 18.7) -> (9, 20.7) centre (9, 19.7) ccw
  line L31 (9, 18.7) -> (-9, 18.7)
  arc A14 (-9, 20.7) -> (-9, 18.7) centre (-9, 19.7) ccw
  line L32 (-9, 20.7) -> (9, 20.7)
  line L33 (8.1652, 14.7) -> (-8.1652, 14.7)
  arc A15 (-8.1652, 16.7) -> (-8.1652, 14.7) centre (-8.1652, 15.7) ccw
  line L34 (-8.1652, 16.7) -> (8.1652, 16.7)
  arc A16 (8.1652, 14.7) -> (8.1652, 16.7) centre (8.1652, 15.7) ccw
  arc A17 (-102.9, 20.7) -> (-102.9, 18.7) centre (-102.9, 19.7) ccw
  line L35 (-102.9, 20.7) -> (-84.9, 20.7)
  arc A18 (-84.9, 18.7) -> (-84.9, 20.7) centre (-84.9, 19.7) ccw
  line L36 (-84.9, 18.7) -> (-102.9, 18.7)
  arc A19 (-98.9, 28.7) -> (-98.9004, 26.7) centre (-98.9, 27.7) ccw
  line L37 (-98.9, 28.7) -> (-88.9, 28.7)
  arc A20 (-88.8996, 26.7) -> (-88.9, 28.7) centre (-88.9, 27.7) ccw
  line L38 (-88.8996, 26.7) -> (-98.9004, 26.7)
  arc A21 (-102.0652, 24.7) -> (-102.0652, 22.7) centre (-102.0652, 23.7) ccw
  line L39 (-102.0652, 24.7) -> (-85.7348, 24.7)
  arc A22 (-85.7348, 22.7) -> (-85.7348, 24.7) centre (-85.7348, 23.7) ccw
  line L40 (-85.7348, 22.7) -> (-102.0652, 22.7)
  line L41 (-85.7348, 14.7) -> (-102.0652, 14.7)
  arc A23 (-102.0652, 16.7) -> (-102.0652, 14.7) centre (-102.0652, 15.7) ccw
  line L42 (-102.0652, 16.7) -> (-85.7348, 16.7)
  arc A24 (-85.7348, 14.7) -> (-85.7348, 16.7) centre (-85.7348, 15.7) ccw
  line L43 (-98.8996, 12.7) -> (-88.8996, 12.7)
  arc A25 (-88.9, 10.7) -> (-88.8996, 12.7) centre (-88.9, 11.7) ccw
  line L44 (-88.9, 10.7) -> (-98.9, 10.7)
  arc A26 (-98.8996, 12.7) -> (-98.9, 10.7) centre (-98.9, 11.7) ccw
  arc A27 (-46.45, -79.6) -> (-47.45, -79.6) centre (-46.95, -79.6) ccw
  line L45 (-46.45, -79.6) -> (-45.65, -79.6)
  arc A28 (-45.65, -80.6) -> (-45.65, -79.6) centre (-45.65, -80.1) ccw
  line L46 (-45.65, -80.6) -> (-46.45, -80.6)
  arc A29 (-47.45, -80.6) -> (-46.45, -80.6) centre (-46.95, -80.6) ccw
  line L47 (-47.45, -80.6) -> (-48.25, -80.6)
  arc A30 (-48.25, -79.6) -> (-48.25, -80.6) centre (-48.25, -80.1) ccw
  line L48 (-48.25, -79.6) -> (-47.45, -79.6)
  circle A31 centre (-110.15, -48.95) radius 3.85
  circle A32 centre (-117.65, -41.45) radius 3.85
  circle A33 centre (-102.65, -41.45) radius 3.85
  circle A34 centre (-110.15, -33.95) radius 3.85
  circle A35 centre (-117.6453, -56.4453) radius 2.35
  circle A36 centre (-102.6547, -56.4453) radius 2.35
  line L49 (0, 4.1) -> (0, -75.1)
  line L50 (0, -75.1) -> (-93.9, -75.1)
  line L51 (-93.9, -75.1) -> (-93.9, 4.1)
  line L52 (-93.9, 4.1) -> (0, 4.1)
  line L53 (15.4643, 29.0958) -> (16.7087, 27.9725)
  line L54 (15.9888, 31.4975) -> (15.9888, 32.8)
  line L55 (15.9888, 32.8) -> (17.8764, 30.7591)
  arc A37 (16.2174, 28.8586) -> (15.4643, 29.0958) centre (16.1, 29.8) ccw
  arc A38 (15.9888, 31.4975) -> (17.8764, 30.7591) centre (16.1, 29) ccw
  line L56 (16.5461, 27.7924) -> (16.7087, 27.9725)
  line L57 (17.0072, 27.998) -> (16.4927, 27.4281)
  line L58 (16.4927, 27.4281) -> (15.2, 27.4281)
  line L59 (15.8651, 28.0068) -> (16.5461, 27.7924)
  line L60 (15.2, 27.4281) -> (15.6347, 27.9403)
  arc A39 (15.8651, 28.0068) -> (15.6347, 27.9403) centre (15.8, 27.8) ccw
  line L61 (17.0072, 27.998) -> (17.0653, 28.0624)
  line L62 (17.0653, 28.0624) -> (16.2174, 28.8586)
  constraint tangent L53 A37
  constraint coincident L0 L54.end
  constraint perpendicular L0 L54
  constraint perpendicular L53 L56
  constraint horizontal L58
  constraint tangent L59 A39
  constraint tangent L60 A39
extrude "Extrude76" cut sketch "icon2" against normal blind 0.8 contours L54 L55 A38 bodies 3
sketch "Sketch91" plane through (-2, 0, 0) normal (-1, 0, 0) x (0, -1, 0)
  line L0 (-24.9, 13.6) -> (-24.9, 14.6)
  line L1 (-24.9, 14.6) -> (-85.1, 14.6)
  line L2 (-85.1, 14.6) -> (-85.1, 10)
  line L3 (-85.1, 10) -> (-77.2, 10)
  line L4 (-77.2, 10) -> (-77.2, 4)
  line L5 (-77.2, 4) -> (-0.9, 4)
  line L6 (-0.9, 4) -> (-0.9, 13.6)
  line L7 (-0.9, 13.6) -> (-1.9, 13.6)
  line L8 (-1.9, 13.6) -> (-1.9, 14.6)
  line L9 (-1.9, 14.6) -> (-6.9, 14.6)
  line L10 (-6.9, 14.6) -> (-6.9, 13.6)
  line L11 (-6.9, 13.6) -> (-7.9, 13.6)
  line L12 (-7.9, 13.6) -> (-7.9, 14.6)
  line L13 (-7.9, 14.6) -> (-12.9, 14.6)
  line L14 (-12.9, 14.6) -> (-12.9, 13.6)
  line L15 (-12.9, 13.6) -> (-13.9, 13.6)
  line L16 (-13.9, 13.6) -> (-13.9, 14.6)
  line L17 (-13.9, 14.6) -> (-18.9, 14.6)
  line L18 (-18.9, 14.6) -> (-18.9, 13.6)
  line L19 (-18.9, 13.6) -> (-24.9, 13.6)
  line L20 (-75.1, 4) -> (-71.1, 4)
  line L21 (-77.2, 4) -> (-77.2, 13.6)
  line L22 (-71.1, 4) -> (-27.1, 4)
  line L23 (-27.1, 4) -> (-27.1, 6)
  line L24 (-71.1, 4) -> (-71.1, 6)
  line L25 (-71.1, 6) -> (-27.1, 6)
  point P0 (-75.1, 4)
  dimension "d626" = 4
  dimension "d627" = 44
  dimension "d628" = 2
  dimension "d629" = 2
  constraint coincident P0 L20.start
  constraint parallel L5 L20
  constraint perpendicular L21 L22
  constraint perpendicular L5 L23
  constraint perpendicular L22 L24
  measures "d626" distance of P0 L20.end
  measures "d627" distance of L20.end L22.end
  measures "d628" distance of L22.end L23.end
  measures "d629" distance of L20.end L24.end
extrude "Extrude77" cut sketch "Sketch91" against normal blind 97.9 contours L5 L22 L23 L24 L25 bodies 3
sketch "Sketch92" plane through (0, 0, 15.6) normal (0, 0, 1) x (-1, 0, 0)
  line L0 (0, 4.1) -> (0, -75.1)
  line L1 (0, -75.1) -> (-93.9, -75.1)
  line L2 (-93.9, -75.1) -> (-93.9, 4.1)
  line L3 (-93.9, 4.1) -> (0, 4.1)
  circle A0 centre (-102.6547, -56.4453) radius 2.35
  circle A1 centre (-117.6453, -56.4453) radius 2.35
  circle A2 centre (-110.15, -33.95) radius 3.85
  circle A3 centre (-102.65, -41.45) radius 3.85
  circle A4 centre (-117.65, -41.45) radius 3.85
  circle A5 centre (-110.15, -48.95) radius 3.85
  arc A6 (-46.45, -79.6) -> (-47.45, -79.6) centre (-46.95, -79.6) ccw
  line L4 (-46.45, -79.6) -> (-45.65, -79.6)
  arc A7 (-45.65, -80.6) -> (-45.65, -79.6) centre (-45.65, -80.1) ccw
  line L5 (-45.65, -80.6) -> (-46.45, -80.6)
  arc A8 (-47.45, -80.6) -> (-46.45, -80.6) centre (-46.95, -80.6) ccw
  line L6 (-47.45, -80.6) -> (-48.25, -80.6)
  arc A9 (-48.25, -79.6) -> (-48.25, -80.6) centre (-48.25, -80.1) ccw
  line L7 (-48.25, -79.6) -> (-47.45, -79.6)
  line L8 (-98.8996, 12.7) -> (-88.8996, 12.7)
  arc A10 (-88.9, 10.7) -> (-88.8996, 12.7) centre (-88.9, 11.7) ccw
  line L9 (-88.9, 10.7) -> (-98.9, 10.7)
  arc A11 (-98.8996, 12.7) -> (-98.9, 10.7) centre (-98.9, 11.7) ccw
  line L10 (-85.7348, 14.7) -> (-102.0652, 14.7)
  arc A12 (-102.0652, 16.7) -> (-102.0652, 14.7) centre (-102.0652, 15.7) ccw
  line L11 (-102.0652, 16.7) -> (-85.7348, 16.7)
  arc A13 (-85.7348, 14.7) -> (-85.7348, 16.7) centre (-85.7348, 15.7) ccw
  arc A14 (-102.0652, 24.7) -> (-102.0652, 22.7) centre (-102.0652, 23.7) ccw
  line L12 (-102.0652, 24.7) -> (-85.7348, 24.7)
  arc A15 (-85.7348, 22.7) -> (-85.7348, 24.7) centre (-85.7348, 23.7) ccw
  line L13 (-85.7348, 22.7) -> (-102.0652, 22.7)
  arc A16 (-98.9, 28.7) -> (-98.9004, 26.7) centre (-98.9, 27.7) ccw
  line L14 (-98.9, 28.7) -> (-88.9, 28.7)
  arc A17 (-88.8996, 26.7) -> (-88.9, 28.7) centre (-88.9, 27.7) ccw
  line L15 (-88.8996, 26.7) -> (-98.9004, 26.7)
  arc A18 (-102.9, 20.7) -> (-102.9, 18.7) centre (-102.9, 19.7) ccw
  line L16 (-102.9, 20.7) -> (-84.9, 20.7)
  arc A19 (-84.9, 18.7) -> (-84.9, 20.7) centre (-84.9, 19.7) ccw
  line L17 (-84.9, 18.7) -> (-102.9, 18.7)
  line L18 (8.1652, 14.7) -> (-8.1652, 14.7)
  arc A20 (-8.1652, 16.7) -> (-8.1652, 14.7) centre (-8.1652, 15.7) ccw
  line L19 (-8.1652, 16.7) -> (8.1652, 16.7)
  arc A21 (8.1652, 14.7) -> (8.1652, 16.7) centre (8.1652, 15.7) ccw
  arc A22 (9, 18.7) -> (9, 20.7) centre (9, 19.7) ccw
  line L20 (9, 18.7) -> (-9, 18.7)
  arc A23 (-9, 20.7) -> (-9, 18.7) centre (-9, 19.7) ccw
  line L21 (-9, 20.7) -> (9, 20.7)
  line L22 (-8.1652, 24.7) -> (8.1652, 24.7)
  arc A24 (8.1652, 22.7) -> (8.1652, 24.7) centre (8.1652, 23.7) ccw
  line L23 (8.1652, 22.7) -> (-8.1652, 22.7)
  arc A25 (-8.1652, 24.7) -> (-8.1652, 22.7) centre (-8.1652, 23.7) ccw
  arc A26 (5.0004, 26.7) -> (5, 28.7) centre (5, 27.7) ccw
  line L24 (5.0004, 26.7) -> (-4.9996, 26.7)
  arc A27 (-5, 28.7) -> (-4.9996, 26.7) centre (-5, 27.7) ccw
  line L25 (-5, 28.7) -> (5, 28.7)
  arc A28 (5, 10.7) -> (5.0004, 12.7) centre (5, 11.7) ccw
  line L26 (5, 10.7) -> (-5, 10.7)
  arc A29 (-5.0004, 12.7) -> (-5, 10.7) centre (-5, 11.7) ccw
  line L27 (-5.0004, 12.7) -> (5.0004, 12.7)
  line L28 (-34.2, 32.4) -> (-34.2, 30.4)
  line L29 (-34.2, 30.4) -> (-27.2, 30.4)
  line L30 (-27.2, 30.4) -> (-27.2, 10)
  arc A30 (-29.2, 8) -> (-27.2, 10) centre (-29.2, 10) ccw
  line L31 (-29.2, 8) -> (-64.7, 8)
  arc A31 (-66.7, 10) -> (-64.7, 8) centre (-64.7, 10) ccw
  line L32 (-66.7, 10) -> (-66.7, 30.4)
  line L33 (-66.7, 30.4) -> (-59.7, 30.4)
  line L34 (-59.7, 30.4) -> (-59.7, 32.4)
  line L35 (-59.7, 32.4) -> (-34.2, 32.4)
  line L36 (13, -32.2) -> (19.5, -32.2)
  line L37 (19.5, -32.2) -> (19.5, -38.2)
  line L38 (19.5, -38.2) -> (25.5, -38.2)
  line L39 (25.5, -38.2) -> (25.5, -44.7)
  line L40 (25.5, -44.7) -> (19.5, -44.7)
  line L41 (19.5, -44.7) -> (19.5, -50.7)
  line L42 (19.5, -50.7) -> (13, -50.7)
  line L43 (13, -50.7) -> (13, -44.7)
  line L44 (13, -44.7) -> (7, -44.7)
  line L45 (7, -44.7) -> (7, -38.2)
  line L46 (7, -38.2) -> (13, -38.2)
  line L47 (13, -38.2) -> (13, -32.2)
  line L48 (29.1144, 32.8) -> (15.9888, 32.8)
  line L49 (15.9888, 32.8) -> (17.8764, 30.7591)
  arc A32 (15.9888, 31.4975) -> (17.8764, 30.7591) centre (16.1, 29) ccw
  line L50 (15.9888, 31.4975) -> (15.9888, 32.8)
  line L51 (15.9888, 32.8) -> (-123.0144, 32.8)
  arc A33 (-123.0144, 32.8) -> (-126.4, 25.3) centre (-116.4, 25.3) ccw
  line L52 (-126.4, 25.3) -> (-126.4, -65.1)
  arc A34 (-126.4, -65.1) -> (-106.4, -85.1) centre (-106.4, -65.1) ccw
  line L53 (-106.4, -85.1) -> (12.5, -85.1)
  arc A35 (12.5, -85.1) -> (32.5, -65.1) centre (12.5, -65.1) ccw
  line L54 (32.5, -65.1) -> (32.5, -25.2)
  line L55 (32.5, -25.2) -> (32.5, 25.3)
  arc A36 (32.5, 25.3) -> (29.1144, 32.8) centre (22.5, 25.3) ccw
  circle A37 centre (10.8119, -62.3239) radius 1.5
  circle A38 centre (-110.15, -48.95) radius 3.85
  circle A39 centre (-117.65, -41.45) radius 3.85
  circle A40 centre (-110.15, -33.95) radius 3.85
  circle A41 centre (-102.65, -41.45) radius 3.85
  circle A42 centre (-102.6547, -56.4453) radius 2.35
  circle A43 centre (-117.6453, -56.4453) radius 2.35
  point P0 (-105.0047, -56.4453)
  point P1 (-119.9953, -56.4453)
  constraint concentric A5 A38
  constraint concentric A4 A39
  constraint concentric A2 A40
  constraint concentric A3 A41
  constraint concentric A0 A42
  constraint coincident A42 P0
  constraint concentric A1 A43
  constraint coincident A43 P1
extrude "Extrude78" cut sketch "Sketch92" against normal blind 2 contours A0 A42 | A1 A43 | A2 A40 | A3 A41 | A4 A39 | A5 A38 bodies 3
fillet "Fillet3" radius 1 8 edges at (-31.6144, -29.4144, 15.6) (-32.5, -0.05, 15.6) (-32.5, 45.15, 15.6) (-26.6421, 79.2421, 15.6) (46.95, 85.1, 15.6) (120.5421, 79.2421, 15.6) (126.4, 19.9, 15.6) (125.5144, -29.4144, 15.6) on bodies 3